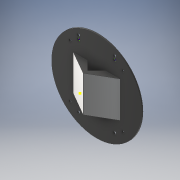
# Autodesk Inventor part: Mirror Mount
Saved by Autodesk Inventor 2018 (Build 220112000, 112)
## iProperties
Created: 2018-08-30
Part Number: Mirror Mount
Material: Acetal Resin, Black
Document SubType Name: Modeling
Designer: matth
Density: 1.425 g/cm^3
Appearance: Smooth - Black
Author: matth
Autodesk Inventor part; units mm, degrees
ref_plane "YZ Plane" through (0, 0, 0) normal (1, 0, 0) x (0, 1, 0)
ref_plane "XZ Plane" through (0, 0, 0) normal (0, 1, 0) x (-1, 0, 0)
ref_plane "XY Plane" through (0, 0, 0) normal (0, 0, 1) x (1, 0, 0)
ref_plane "Work Plane3" through (-4.3301, 20, -20) normal (0, 1, 0) x (1, 0, 0)
sketch "Sketch4" plane through (-4.3301, 20, -20) normal (0, 1, 0) x (1, 0, 0)
  circle A0 centre (4.3301, -20) radius 50
  dimension "d16" = 100
  constraints: 1 centre point, 1 coincident
  measures "d16" diameter of A0
extrude "Extrusion4" add sketch "Sketch4" along normal blind 1.5
sketch "Sketch9" plane through (0, 0, 0) normal (0, 0, 1) x (1, 0, 0)
  line L0 (50, 21.5) -> (-50, 21.5) projected
  line L1 (50, 21.5) -> (43, 21.5)
  line L2 (50, 21.5) -> (50, 26.5)
  line L3 (50, 26.5) -> (48, 26.5)
  line L4 (48, 26.5) -> (43, 21.5)
  line L5 (0, 21.5) -> (0, 37.2)
  point P0 (0, 0)
  dimension "d27" = 7
  dimension "d28" = 5
  dimension "d29" = 2
  constraints: 10 end point, 2 vertical, 1 midpoint, 1 perpendicular, 1 point on line
  measures "d27" distance of L0.start L1.end
  measures "d28" distance of L0.start L2.end
  measures "d29" distance of L2.end L3.end
revolve "Revolution1" add sketch "Sketch9" angle 360 about axis through (0, 21.5, 0) along (0, 1, 0)
ref_plane "Work Plane2" through (0, 21.5, 0) normal (0, 1, 0) x (1, 0, 0)
sketch "Sketch12" plane through (0, 21.5, 0) normal (0, 1, 0) x (1, 0, 0)
  line L0 (0, 0) -> (20, 0)
  line L1 (20, 0) -> (20, -35)
  line L2 (20, -35) -> (-20, -35)
  line L3 (-20, -35) -> (-20, 35)
  line L4 (-20, 35) -> (20, 35)
  line L5 (20, 35) -> (20, -35)
  circle A0 centre (20, 35) radius 1.75
  circle A1 centre (-20, 35) radius 1.75
  circle A2 centre (-20, -35) radius 1.75
  circle A3 centre (20, -35) radius 1.75
  dimension "d47" = 20
  dimension "d48" = 35
  dimension "d49" = 40
  dimension "d50" = 70
  dimension "d51" = 3.5
  dimension "d52" = 3.5
  dimension "d53" = 3.5
  dimension "d54" = 3.5
  constraints: 12 end point, 4 centre point, 4 coincident, 2 horizontal, 2 parallel, 2 perpendicular
  measures "d47" distance of L0.start L0.end
  measures "d48" distance of L0.end L1.end
  measures "d49" distance of L3.end L4.end
  measures "d50" distance of L2.end L3.end
  measures "d51" diameter of A0
  measures "d52" diameter of A1
  measures "d53" diameter of A2
  measures "d54" diameter of A3
extrude "Extrusion6" cut sketch "Sketch12" against normal blind 1.5 contours A3 L2 L1 | L1 L2 A3 | A0 L4 L5 | L5 L4 A0 | A2 L3 L2 | L2 L3 A2 | A1 L3 L4 | L4 L3 A1
sketch "Sketch13" plane through (0, 0, 0) normal (0, 0, 1) x (1, 0, 0)
  line L0 (0, 0) -> (25, 0) construction
  line L1 (-50, 20) -> (50, 20) projected
  line L2 (0, 7.5) -> (-21.6506, 20)
  line L3 (0, 7.5) -> (21.6506, 20)
  line L4 (0, 7.5) -> (25, 7.5) construction
  line L5 (21.6506, 20) -> (-21.6506, 20)
  line L6 (0, 7.5) -> (0, 12.5)
  line L7 (0, 20) -> (-5, 20)
  line L8 (-5, 20) -> (0, 12.5)
  line L9 (0, 20) -> (5, 20)
  line L10 (5, 20) -> (0, 12.5)
  dimension "d60" = 25
  dimension "d61" = 30
  dimension "d62" = 5
  dimension "d63" = 5
  dimension "d64" = 5
  constraints: 20 end point, 3 point on line, 2 horizontal, 1 collinear, 1 equal length, 1 midpoint, 1 perpendicular
  measures "d60" distance of L2.start L3.end
  measures "d61" angle of L4 L3
  measures "d62" distance of L2.start L6.end
  measures "d63" distance of L7.start L7.end
  measures "d64" distance of L7.start L9.end
extrude "Extrusion7" add sketch "Sketch13" along normal mid plane 40 contours L1 L8 L6 L2 | L6 L10 L1 L3
sketch "Sketch16" plane through (0, 0, 20) normal (0, 0, 1) x (1, 0, 0)
  line L0 (-50, 20) -> (50, 20) projected
  line L1 (0, 20) -> (0, 5)
  line L2 (0, 5) -> (23.8952, 18.7959)
  line L3 (23.8952, 18.7959) -> (25.9808, 20)
  line L4 (25.9808, 20) -> (-25.9812, 20)
  line L5 (-25.9812, 20) -> (0, 5)
  point P0 (0, 0)
  dimension "d67" = 15
  dimension "d68" = 60
  dimension "d69" = 51.962
  constraints: 10 end point, 3 point on line, 1 midpoint, 1 vertical
  measures "d67" distance of L1.start L1.end
  measures "d68" angle of L2 L1
  measures "d69" distance of L3.end L4.end
extrude "Extrusion8" add sketch "Sketch16" against normal blind 40
sketch "Sketch17" plane through (0, 0, 20) normal (0, 0, 1) x (1, 0, 0)
  line L0 (0, 5) -> (-25.9812, 20) projected
  line L1 (0, 5) -> (0, 10)
  line L2 (0, 10) -> (6.8298, 16.8298)
  line L3 (6.8298, 16.8298) -> (10, 20)
  line L4 (-50, 20) -> (50, 20) projected
  line L5 (10, 20) -> (-10, 20)
  line L6 (-10, 20) -> (0, 10)
  point P0 (0, 0)
  dimension "d72" = 5
  dimension "d73" = 135
  dimension "d74" = 20
  constraints: 10 end point, 3 point on line, 1 vertical
  measures "d72" distance of L0.start L1.end
  measures "d73" angle of L1 L2
  measures "d74" distance of L3.end L5.end
extrude "Extrusion9" cut sketch "Sketch17" against normal blind 40 contours L6 L4 L3 L2
sketch "Sketch18" plane through (0, 20, 0) normal (0, -1, 0) x (1, 0, 0)
  line L0 (0, 0) -> (-35.3553, 35.3553)
  circle A0 centre (0, 0) radius 50 projected
  line L1 (0, 0) -> (50, 0) construction
  line L2 (0, 0) -> (35.3553, 35.3553)
  line L3 (0, 0) -> (50, 0) construction
  line L4 (0, 0) -> (-35.3553, -35.3553)
  line L5 (0, 0) -> (50, 0) construction
  line L6 (0, 0) -> (35.3553, -35.3553)
  line L7 (0, 0) -> (50, 0) construction
  circle A1 centre (0, 0) radius 43 projected
  line L8 (-30.4056, 30.4056) -> (-29.3449, 29.3449)
  line L9 (30.4056, 30.4056) -> (29.3449, 29.3449)
  line L10 (30.4056, -30.4056) -> (29.3449, -29.3449)
  line L11 (-30.4056, -30.4056) -> (-29.3449, -29.3449)
  circle A2 centre (-29.3449, -29.3449) radius 1.5
  circle A3 centre (29.3449, -29.3449) radius 1.5
  circle A4 centre (-29.3449, 29.3449) radius 1.5
  circle A5 centre (29.3449, 29.3449) radius 1.5
  dimension "d77" = 135
  dimension "d78" = 45
  dimension "d79" = 135
  dimension "d80" = 45
  dimension "d81" = 1.5
  dimension "d82" = 1.5
  dimension "d83" = 1.5
  dimension "d84" = 1.5
  constraints: 24 end point, 8 point on circle, 8 point on line, 4 coincident, 4 equal length, 4 horizontal, 12 other
  measures "d77" angle of L1 L0
  measures "d78" angle of L3 L2
  measures "d79" angle of L4 L5
  measures "d80" angle of L6 L7
  measures "d81" distance of L8.start L8.end
  measures "d82" distance of L9.start L9.end
  measures "d83" distance of L10.start L10.end
  measures "d84" distance of L11.start L11.end
extrude "Extrusion10" cut sketch "Sketch18" against normal blind 40 contours A4 L0 | L0 A4 | A5 L2 | L2 A5 | A2 L4 | L4 A2 | A3 L6 | L6 A3
sketch "Sketch20" plane through (-4.3301, 21.5, -20) normal (0, 1, 0) x (1, 0, 0)
  circle A0 centre (-15.6699, 15) radius 1.75 projected
  circle A1 centre (-15.6699, 15) radius 3.5
  circle A2 centre (24.3301, 15) radius 1.75 projected
  circle A3 centre (24.3301, 15) radius 3.5
  circle A4 centre (24.3301, -55) radius 1.75 projected
  circle A5 centre (24.3301, -55) radius 3.5
  circle A6 centre (-15.6699, -55) radius 1.75 projected
  circle A7 centre (-15.6699, -55) radius 3.5
  point P0 (4.3301, -20)
  dimension "d87" = 7
  dimension "d88" = 7
  dimension "d89" = 7
  dimension "d90" = 7
  constraints: 4 centre point, 4 coincident
  measures "d87" diameter of A1
  measures "d88" diameter of A3
  measures "d89" diameter of A5
  measures "d90" diameter of A7
extrude "Extrusion11" cut sketch "Sketch20" along normal blind 10
sketch "Sketch21" plane through (-4.3301, 21.5, -20) normal (0, 1, 0) x (1, 0, 0)
  circle A0 centre (4.3301, -20) radius 67.7461
  constraints: 1 centre point, 1 coincident
extrude "Extrusion12" cut sketch "Sketch21" along normal blind 10
sketch "Sketch22" plane through (0, 5, -20) normal (0.5, -0.8660254, 0) x (0.8660254, 0.5, 0)
  point P0 (-2.5, 20)
sketch "Sketch23" plane through (0, 21.5, 0) normal (0, 1, 0) x (1, 0, 0)
  circle A0 centre (20, -35) radius 1.75 projected
  line L0 (20, -35) -> (20, -39)
  circle A1 centre (-20, -35) radius 1.75 projected
  line L1 (-20, -35) -> (-20, -39)
  circle A2 centre (20, -39) radius 1.75
  circle A3 centre (-20, -39) radius 1.75
  point P0 (0, 0)
  dimension "d95" = 4
  dimension "d96" = 4
  dimension "d97" = 3.5
  dimension "d98" = 3.5
  constraints: 4 end point, 2 centre point, 2 coincident, 2 vertical
  measures "d95" distance of L0.start L0.end
  measures "d96" distance of L1.start L1.end
  measures "d97" diameter of A2
  measures "d98" diameter of A3
extrude "Extrusion13" cut sketch "Sketch23" against normal blind 10 contours A2 | A3
sketch "Sketch24" plane through (0, 21.5, 0) normal (0, 1, 0) x (1, 0, 0)
  circle A0 centre (20, -35) radius 1.75 projected
  circle A1 centre (20, -35) radius 1.75
  circle A2 centre (-20, -35) radius 1.75 projected
  circle A3 centre (-20, -35) radius 1.75
  point P0 (0, 0)
  constraints: 2 centre point, 2 coincident
body "Solid1"
